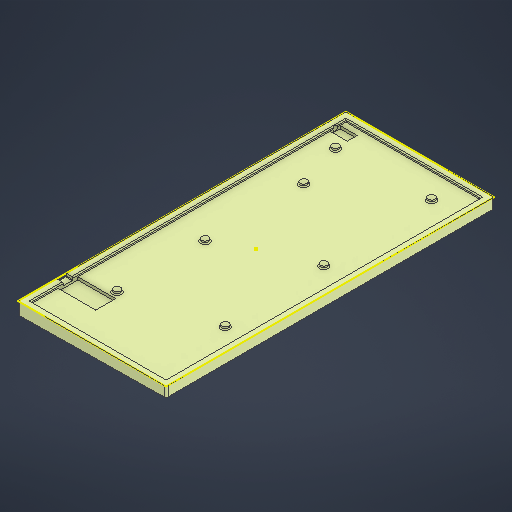
# Autodesk Inventor part: Keyboard_Tray
Saved by Autodesk Inventor 2026.1 (Build 301233000, 233)
## iProperties
Created: 2025-11-08
Part Number: Keyboard_Tray
Material: Generic
Document SubType Name: Modeling
Designer: avani
Density: 1 g/cm^3
Appearance: Default
Author: avani
Autodesk Inventor part; units mm, degrees
ref_plane "YZ Plane" through (0, 0, 0) normal (1, 0, 0) x (0, 1, 0)
ref_plane "XZ Plane" through (0, 0, 0) normal (0, 1, 0) x (-1, 0, 0)
ref_plane "XY Plane" through (0, 0, 0) normal (0, 0, 1) x (1, 0, 0)
sketch "Sketch1" plane through (0, 0, 0) normal (0, 1, 0) x (-1, 0, 0)
  line L0 (-67.875, 158.365) -> (67.875, 158.365)
  line L1 (67.875, 158.365) -> (67.875, -158.365)
  line L2 (67.875, -158.365) -> (-67.875, -158.365)
  line L3 (-67.875, -158.365) -> (-67.875, 158.365)
  line L4 (-67.875, 158.365) -> (67.875, -158.365) construction
  line L5 (67.875, 158.365) -> (-67.875, -158.365) construction
  line L6 (-74.5, 165) -> (74.5, 165)
  line L7 (74.5, 165) -> (74.5, -165)
  line L8 (74.5, -165) -> (-74.5, -165)
  line L9 (-74.5, -165) -> (-74.5, 165)
  line L10 (-74.5, 165) -> (74.5, -165) construction
  line L11 (74.5, 165) -> (-74.5, -165) construction
  point P0 (0, 0)
  dimension "d0" = 135.75
  dimension "d1" = 316.73
  dimension "d2" = 149
  dimension "d3" = 330
  constraints: 24 end point, 4 midpoint, 4 parallel, 2 horizontal, 2 perpendicular
  measures "d0" distance of L1.end L2.end
  measures "d1" distance of L0.end L1.end
  measures "d2" distance of L7.end L8.end
  measures "d3" distance of L6.end L7.end
extrude "Extrusion1" add sketch "Sketch1" against normal blind 12 contours L0 L1 L2 L3 | L6 L7 L8 L9
sketch "Sketch2" plane through (0, 0, 0) normal (0, 1, 0) x (1, 0, 0)
  line L0 (-74.5, -165) -> (-74.5, 165) projected
  line L1 (-74.5, 165) -> (74.5, 165) projected
  line L2 (74.5, 165) -> (74.5, -165) projected
  line L3 (74.5, -165) -> (-74.5, -165) projected
  point P0 (0, 0)
sketch "Sketch3" plane through (0, 0, 0) normal (0, 1, 0) x (1, 0, 0)
  line L0 (-67.875, -158.365) -> (67.875, -158.365)
  line L1 (67.875, -158.365) -> (67.875, 158.365)
  line L2 (67.875, 158.365) -> (-67.875, 158.365)
  line L3 (-67.875, 158.365) -> (-67.875, -158.365)
  line L4 (-67.875, -158.365) -> (67.875, 158.365) construction
  line L5 (67.875, -158.365) -> (-67.875, 158.365) construction
  point P0 (0, 0)
  dimension "d6" = 135.75
  dimension "d7" = 316.73
  constraints: 12 end point, 2 midpoint, 2 parallel, 1 horizontal, 1 perpendicular
  measures "d6" distance of L2.end L1.end
  measures "d7" distance of L1.end L0.end
extrude "Extrusion2" cut sketch "Sketch3" against normal blind 2.4
chamfer "Chamfer1" distance 1 angle 45 4 edges at (-67.875, 0, 0) (0, 0, -158.365) (67.875, 0, 0) (0, 0, 158.365)
fillet "Fillet1" radius 1 4 edges at (-67.875, -1.7, -158.365) (67.875, -1.7, -158.365) (67.875, -1.7, 158.365) (-67.875, -1.7, 158.365)
sketch "Sketch5" plane through (0, -2.4, 0) normal (0, 1, 0) x (1, 0, 0)
  circle A0 centre (-35.008, -104.7817) radius 3.5
  circle A1 centre (43.1604, 133.5) radius 3.5
  circle A2 centre (50, -80.8806) radius 3.5
  circle A3 centre (-50, 130) radius 3.5
  circle A4 centre (-35.008, -16.2037) radius 3.5
  circle A5 centre (46.5, 21.7724) radius 3.5
  circle A6 centre (-35.008, 82.9775) radius 3.5
  point P0 (0, 0)
  dimension "d14" = 7
  dimension "d15" = 7
  dimension "d16" = 7
  dimension "d17" = 7
  dimension "d18" = 7
  dimension "d19" = 7
  dimension "d44" = 7
  constraints: 7 centre point
  measures "d14" diameter of A0
  measures "d15" diameter of A1
  measures "d16" diameter of A2
  measures "d17" diameter of A3
  measures "d18" diameter of A4
  measures "d19" diameter of A5
  measures "d44" diameter of A6
extrude "Extrusion3" add sketch "Sketch5" along normal blind 2.4
fillet "Fillet2" radius 1 7 edges at (-38.508, -2.4, 104.7817) (46.5, -2.4, 80.8806) (-38.508, -2.4, 16.2037) (43, -2.4, -21.7724) (39.6604, -2.4, -133.5) (-53.5, -2.4, -130) (-38.508, -2.4, -82.9775)
sketch "Sketch6" plane through (0, 0, 0) normal (0, 1, 0) x (1, 0, 0)
  line L0 (-74.5, -165) -> (-74.5, 165) projected
  line L1 (-74.5, 144.365) -> (-50.5, 144.365)
  line L2 (-50.5, 144.365) -> (-50.5, 150.465)
  line L3 (-50.5, 150.465) -> (-74.5, 150.465)
  line L4 (-74.5, 150.465) -> (-74.5, 144.365)
  line L5 (74.5, 165) -> (-74.5, 165) projected
  line L6 (-67.8251, 144.365) -> (-50.5, 144.365)
  line L7 (-50.5, 144.365) -> (-50.5, 152.365)
  line L8 (-50.5, 152.365) -> (-67.8251, 152.365)
  line L9 (-67.8251, 152.365) -> (-67.8251, 144.365)
  line L10 (-50.5, 152.365) -> (-67.8251, 152.365)
  line L11 (-67.8251, 152.365) -> (-67.8251, 142.365)
  line L12 (-67.8251, 142.365) -> (-50.5, 142.365)
  line L13 (-50.5, 142.365) -> (-50.5, 152.365)
  line L14 (-67.875, -157.365) -> (-67.875, 157.365) projected
  line L15 (-67.875, -131.365) -> (-29.875, -131.365)
  line L16 (-29.875, -131.365) -> (-29.875, -111.365)
  line L17 (-29.875, -111.365) -> (-67.875, -111.365)
  line L18 (-67.875, -111.365) -> (-67.875, -131.365)
  line L19 (66.875, -158.365) -> (-66.875, -158.365) projected
  line L20 (-66.875, 158.365) -> (66.875, 158.365) projected
  point P0 (0, 0)
  point P1 (-67.8251, 150.465)
  point P2 (-48.875, -131.365)
  dimension "d26" = 6.1
  dimension "d27" = 24
  dimension "d28" = 8
  dimension "d29" = 10
  dimension "d40" = 20
  dimension "d41" = 27
  dimension "d42" = 38
  dimension "d43" = 6
  constraints: 32 end point, 8 parallel, 4 horizontal, 4 perpendicular, 3 point on line, 1 midpoint
  measures "d26" distance between parallel lines of L3 L1
  measures "d27" distance of L1.start L1.end
  measures "d28" distance of L7.end L6.end
  measures "d29" distance of L11.end L10.end
  measures "d40" distance of L15.end L16.end
  measures "d41" distance from line of L19 point (-48.875, -131.365)
  measures "d42" distance between parallel lines of L16 L14
  measures "d43" distance between parallel lines of L8 L20
extrude "Extrusion4" cut sketch "Sketch6" against normal blind 5.2 contours L17 L16 L15 L14 | L9 L3 L2 L1 | L1 L13 L12 L11 | L9 L8 L7 L3
sketch "Sketch7" plane through (-74.5, 0, -165) normal (-1, 0, 0) x (0, 0, 1)
  line L0 (330, -12) -> (0, -12) projected
  line L1 (0, -12) -> (14.3, -12)
  line L2 (14.3, -12) -> (14.3, -5.6744)
  line L3 (14.3, -5.6744) -> (0, -5.6744)
  line L4 (0, -5.6744) -> (0, -12)
  line L5 (5.635, 0) -> (324.365, 0) projected
  line L6 (14.3, -12) -> (20.4, -12)
  line L7 (20.4, -12) -> (20.4, 0)
  line L8 (20.4, 0) -> (14.3, 0)
  line L9 (14.3, 0) -> (14.3, -12)
  circle A0 centre (17.35, -2.6) radius 2.4
  line L10 (330, 0) -> (330, -12) projected
  line L11 (330, -12) -> (291, -12)
  line L12 (291, -12) -> (291, -0.5)
  line L13 (291, 0) -> (330, 0)
  line L14 (330, 0) -> (330, -12)
  line L15 (291, -12) -> (281.5, -12)
  line L16 (281.5, -12) -> (281.5, -0.5)
  line L17 (282, 0) -> (290.5, 0)
  line L18 (291, 0) -> (291, -12)
  line L19 (291, 0) -> (281.5, 0)
  line L20 (281.5, 0) -> (281.5, -2.4)
  line L21 (282, -2.9) -> (290.5, -2.9)
  line L22 (291, -2.4) -> (291, 0)
  arc A1 (290.5, -2.9) -> (291, -2.4) centre (290.5, -2.4) ccw
  arc A2 (291, -0.5) -> (290.5, 0) centre (290.5, -0.5) ccw
  arc A3 (281.5, -2.4) -> (282, -2.9) centre (282, -2.4) ccw
  arc A4 (282, 0) -> (281.5, -0.5) centre (282, -0.5) ccw
  point P0 (165, 0)
  point P1 (17.35, -12)
  point P2 (281.5, -12)
  point P3 (291, -12)
  point P4 (281.5, -2.9)
  point P5 (291, -3)
  point P6 (281.5, -2.4)
  point P7 (281.5, -0.5)
  point P8 (281.5, -0.5)
  dimension "d30" = 14.3
  dimension "d31" = 6.1
  dimension "d34" = 9.4
  dimension "d35" = 4.8
  dimension "d36" = 39
  dimension "d37" = 9.5
  dimension "d38" = 9.1
  dimension "d39" = 0.5
  constraints: 40 end point, 10 parallel, 10 point on line, 8 point on circle, 8 tangent, 5 centre point, 5 horizontal, 5 perpendicular, 3 equal radius, 1 midpoint
  measures "d30" distance of L3.end L2.end
  measures "d31" distance of L8.end L7.end
  measures "d34" distance of point (17.35, -12) A0.centre
  measures "d35" diameter of A0
  measures "d36" distance between parallel lines of L10 L12
  measures "d37" distance between parallel lines of L18 L16
  measures "d38" distance between parallel lines of L0 L21
  measures "d39" radius of A1
extrude "Extrusion5" cut sketch "Sketch7" against normal up to surface contours A1 L21 A3 L16 A4 L5 A2 L12 | A2 L5 L18 | L20 L5 A4 | A0 surface through (-68.375, -0.5, 79.1825) normal (0.7071, 0.7071, 0)
chamfer "Chamfer2" distance 149 distance2 2 1 edges at (74.5, -12, 0) measured on face at (24.8333, -12, 55)
fillet "Fillet3" radius 2 4 edges at (-74.5, -6, 165) (74.5, -5.0003, 165) (74.5, -5.0003, -165) (-74.5, -6, -165)
body "Solid1"
